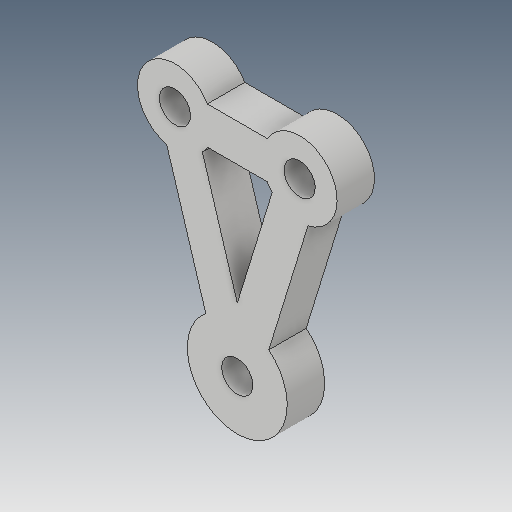
# Autodesk Inventor part: 従動節固定
Saved by Autodesk Inventor 2019.4 (Build 234330000, 330)
## iProperties
Created: 2018-08-30
Part Number: 従動節固定
Material: 一般
Document SubType Name: Modeling
Designer: AzLIer
Density: 1 g/cm^3
Appearance: 既定
Author: AzLIer
Autodesk Inventor part; units mm, degrees
note: some values were not read from the file. Chosen so that the rebuilt part matches the saved one: sketch regions of "押し出し1".
ref_plane "YZ Plane" through (0, 0, 0) normal (1, 0, 0) x (0, 1, 0)
ref_plane "XZ Plane" through (0, 0, 0) normal (0, 1, 0) x (-1, 0, 0)
ref_plane "作業平面1" through (14.45, -5.25, 10.5) normal (0, 0, 1) x (0, 1, 0)
sketch "スケッチ1" plane through (14.45, -5.25, 10.5) normal (0, 0, 1) x (0, 1, 0)
  circle A0 centre (4.8, 4.5) radius 1.25
  circle A1 centre (4.8, 14.5) radius 1.25
  circle A2 centre (4.5, 225.5) radius 1.5 projected
  circle A3 centre (4.5, 201.5) radius 1.5 projected
  line L0 (9, 0) -> (0, 0) projected
  line L1 (9, 0) -> (9, 230) projected
  line L2 (0, 230) -> (9, 230) projected
  line L3 (0, 0) -> (0, 230) projected
  circle A4 centre (-11.4155, 9.5) radius 1.25
  circle A5 centre (4.8, 14.5) radius 4.6
  circle A6 centre (4.8, 4.5) radius 4.6
  circle A7 centre (-11.4155, 9.5) radius 4.25
  line L4 (9.4, 19.1) -> (-15.6655, 19.1)
  line L5 (-15.6655, 19.1) -> (-15.6655, -0.1)
  line L6 (-15.6655, -0.1) -> (9.4, -0.1)
  line L7 (9.4, -0.1) -> (9.4, 19.1)
  point P0 (5.25, 14.45)
  dimension "d0" = 2.5
  dimension "d1" = 9.2
  dimension "d2" = 9.2
  dimension "d3" = 8.5
  dimension "d14" = 2.5
  constraints: 8 end point, 6 centre point, 4 tangent, 2 parallel, 1 coincident, 1 equal radius, 1 horizontal, 1 perpendicular, 2 other
  measures "d0" diameter of A4
  measures "d1" diameter of A5
  measures "d2" diameter of A6
  measures "d3" diameter of A7
  measures "d14" diameter of A0
extrude "押し出し1" add sketch "スケッチ1" along normal blind 3 contours L1 A6 L7 L6 L0 | L0 A6 L1 | A6 L0 | L0 A6 L1 | L1 A6 | A7 | A6 L6 L5 L4 L3 L0 | L0 L3 L4 A5 L1 A6 | L1 A5 L7 A6 | A5 L1 | L1 A5 | A5 L1 L4 L7 | A5 L4 L1
sketch "スケッチ2" plane through (14.45, -5.25, 10.5) normal (0, 0, -1) x (-1, 0, 0)
  circle A0 centre (4.5, 4.8) radius 1.25 projected
  circle A1 centre (14.5, 4.8) radius 1.25 projected
  circle A2 centre (9.5, -11.4155) radius 1.25 projected
  line L0 (-0.1, -15.6655) -> (-0.1, 9.4) projected
  line L1 (-0.1, 9.4) -> (19.1, 9.4) projected
  line L2 (19.1, 9.4) -> (19.1, -15.6655) projected
  line L3 (19.1, -15.6655) -> (-0.1, -15.6655) projected
  circle A3 centre (4.5, 4.8) radius 3
  circle A4 centre (14.5, 4.8) radius 3
  circle A5 centre (9.5, -11.4155) radius 4
  line L4 (4.5, 4.8) -> (9.5, -11.4155) construction
  line L5 (3.0666, 4.358) -> (8.0666, -11.8575)
  line L6 (10.9334, -10.9735) -> (5.9334, 5.242)
  arc A6 (5.9334, 5.242) -> (3.0666, 4.358) centre (4.5, 4.8) ccw
  arc A7 (8.0666, -11.8575) -> (10.9334, -10.9735) centre (9.5, -11.4155) ccw
  line L7 (9.5, -11.4155) -> (14.5, 4.8) construction
  line L8 (10.9334, -11.8575) -> (15.9334, 4.358)
  line L9 (13.0666, 5.242) -> (8.0666, -10.9735)
  arc A8 (8.0666, -10.9735) -> (10.9334, -11.8575) centre (9.5, -11.4155) ccw
  arc A9 (15.9334, 4.358) -> (13.0666, 5.242) centre (14.5, 4.8) ccw
  line L10 (4.5, 4.8) -> (14.5, 4.8) construction
  line L11 (4.5, 3.3) -> (14.5, 3.3)
  line L12 (14.5, 6.3) -> (4.5, 6.3)
  arc A10 (4.5, 6.3) -> (4.5, 3.3) centre (4.5, 4.8) ccw
  arc A11 (14.5, 3.3) -> (14.5, 6.3) centre (14.5, 4.8) ccw
  point P0 (14.45, 5.25)
  point P1 (7, -3.3077)
  point P2 (12, -3.3077)
  point P3 (9.5, 4.8)
  dimension "d6" = 6
  dimension "d7" = 6
  dimension "d8" = 8
  dimension "d9" = 3
  dimension "d10" = 3
  dimension "d11" = 3
  constraints: 24 end point, 12 point on circle, 12 tangent, 9 centre point, 3 coincident, 3 midpoint, 3 parallel, 1 concentric, 1 horizontal
  measures "d6" diameter of A3
  measures "d7" diameter of A4
  measures "d8" diameter of A5
  measures "d9" diameter of A7
  measures "d10" diameter of A9
  measures "d11" diameter of A11
extrude "押し出し2" cut sketch "スケッチ2" against normal blind 10 contours A0 | A1 | A2 | A3 L11 L6 A6 L12 | A3 L12 A4 L11 | L12 A6 L5 A3 | A3 L6 L11 | L5 A10 L11 L6 A3 | A3 L6 L9 A5 L5 | L12 A9 L9 L11 A4 | A4 L8 A9 L12 | A6 L6 L11 A10 | L11 L9 A4 | L5 A7 L8 A5 | A5 L9 A8 L5 | A9 A11 L11 L9 | L9 A4 L8 A5 L6 | L6 A5 L9 | L9 L11 A11 L8 A4 | A5 L6 A7 A8 L9 | A5 L8 A7 L6 keep common part
